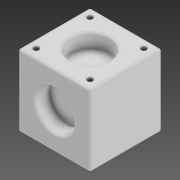
# Autodesk Inventor part: 3 dubbele lagerblok
Saved by Autodesk Inventor 2020 (Build 240168000, 168)
## iProperties
Created: 2020-05-19
Part Number: 3 dubbele lagerblok
Material: Generic
Document SubType Name: Modeling
Designer: stefa
Density: 1 g/cm^3
Appearance: Default
Author: stefa
Autodesk Inventor part; units mm, degrees
ref_plane "YZ Plane" through (0, 0, 0) normal (1, 0, 0) x (0, 1, 0)
ref_plane "XZ Plane" through (0, 0, 0) normal (0, 1, 0) x (-1, 0, 0)
ref_plane "XY Plane" through (0, 0, 0) normal (0, 0, 1) x (1, 0, 0)
sketch "Sketch1" plane through (0, 0, 0) normal (0, 1, 0) x (-1, 0, 0)
  line L0 (-20, 20) -> (20, 20)
  line L1 (20, 20) -> (20, -20)
  line L2 (20, -20) -> (-20, -20)
  line L3 (-20, -20) -> (-20, 20)
  line L4 (-20, 20) -> (20, -20) construction
  line L5 (20, 20) -> (-20, -20) construction
  circle A0 centre (15, 15) radius 1.5
  circle A1 centre (15, -15) radius 1.5
  circle A2 centre (-15, 15) radius 1.5
  circle A3 centre (-15, -15) radius 1.5
  point P0 (0, 0)
  dimension "d1" = 40
  dimension "d10" = 3
  dimension "d11" = 5
  dimension "d14" = 30
  dimension "d17" = 30
  constraints: 12 end point, 4 centre point, 2 horizontal, 2 midpoint, 2 parallel, 2 perpendicular, 1 point on line, 1 vertical, 6 other
  measures "d1" distance of L0.end L1.end
  measures "d10" diameter of A0
  measures "d11" distance from line of L1 A0.centre
  measures "d14" distance of A0.centre A1.centre
  measures "d17" distance of A0.centre A2.centre
extrude "Extrusion1" add sketch "Sketch1" along normal mid plane 40
sketch "Sketch2" plane through (0, 20, 0) normal (0, 1, 0) x (1, 0, 0)
  circle A0 centre (0, 0) radius 11
  dimension "d4" = 22
  constraints: 1 centre point, 1 coincident
  measures "d4" diameter of A0
extrude "Extrusion2" cut sketch "Sketch2" against normal blind 8
sketch "Sketch3" plane through (-20, 20, 20) normal (0, 0, 1) x (1, 0, 0)
  circle A0 centre (20, -20) radius 11
  dimension "d7" = 22
  constraints: 1 centre point, 1 coincident
  measures "d7" diameter of A0
extrude "Extrusion3" cut sketch "Sketch3" against normal blind 8
mirror "Mirror2" about plane through (0, 0, 0) normal (0, 0, 1) of "Extrusion3"
fillet "Fillet1" radius 1 3 edges at (-11, 20, 0) (-11, 0, 20) (-11, 0, -20)
fillet "Fillet2" radius 1 12 edges at (20, 0, 20) (20, 20, 0) (0, 20, 20) (20, 0, -20) (0, 20, -20) (-20, 0, -20) (-20, 20, 0) (-20, 0, 20) (-20, -20, 0) (0, -20, -20) (20, -20, 0) (0, -20, 20)
equation "\"d14\" = d1 - 2 * d11"
equation "\"d17\" = d14"
body "Solid1"
